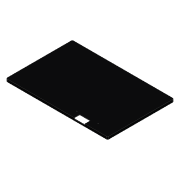
# Autodesk Inventor part: printer floor plate
Saved by Autodesk Inventor 2015 (Build 190159000, 159)
## iProperties
Created: 2018-06-07
Part Number: printer floor plate
Material: Generic
Document SubType Name: Modeling
Designer: Ghassan Yusuf
Density: 1 g/cm^3
Appearance: Default(1)
Author: Ghassan Yusuf
Autodesk Inventor part; units mm, degrees
ref_plane "YZ Plane" through (0, 0, 0) normal (1, 0, 0) x (0, 1, 0)
ref_plane "XZ Plane" through (0, 0, 0) normal (0, 1, 0) x (-1, 0, 0)
ref_plane "XY Plane" through (0, 0, 0) normal (0, 0, 1) x (1, 0, 0)
sketch "Sketch1" plane through (0, 0, 0) normal (0, 0, 1) x (1, 0, 0)
  line L0 (-236.677, 154.5) -> (236.677, 154.5)
  line L1 (236.677, 154.5) -> (236.677, -154.5)
  line L2 (236.677, -154.5) -> (-236.677, -154.5)
  line L3 (-236.677, -154.5) -> (-236.677, 154.5)
  point P0 (0, 0)
  point P1 (0, 154.5)
  point P2 (-236.677, 0)
  dimension "d0" = 473.354
  dimension "d1" = 309
  constraints: 8 end point, 2 midpoint, 2 parallel, 1 horizontal, 1 horizontal alignment, 1 perpendicular, 1 vertical alignment
  measures "d0" distance of L1.end L2.end
  measures "d1" distance of L0.end L1.end
extrude "Extrusion1" add sketch "Sketch1" along normal blind 2
sketch "Sketch2" plane through (0, 0, 2) normal (0, 0, 1) x (1, 0, 0)
  line L0 (-236.677, 154.5) -> (236.677, 154.5)
  line L1 (236.677, 154.5) -> (236.677, -154.5)
  line L2 (236.677, -154.5) -> (-236.677, -154.5)
  line L3 (-236.677, -154.5) -> (-236.677, 154.5)
  line L4 (-234.677, 152.5) -> (234.677, 152.5)
  line L5 (234.677, 152.5) -> (234.677, -152.5)
  line L6 (234.677, -152.5) -> (-234.677, -152.5)
  line L7 (-234.677, -152.5) -> (-234.677, 152.5)
  point P0 (0, 0)
  dimension "d4" = 2
  constraints: 16 end point, 4 parallel, 2 perpendicular, 1 horizontal, 3 other
  measures "d4" distance between parallel lines of L3 L7
extrude "Extrusion2" add sketch "Sketch2" along normal blind 10
fillet "Fillet1" radius 5 8 edges at (236.677, -154.5, 6) (234.677, -152.5, 7) (-236.677, -154.5, 6) (-234.677, -152.5, 7) (-234.677, 152.5, 7) (236.677, 154.5, 6) (234.677, 152.5, 7) (-236.677, 154.5, 6)
sketch "Sketch4" plane through (0, 0, 0) normal (0, 0, -1) x (-1, 0, 0)
  line L0 (-231.677, -154.5) -> (231.677, -154.5)
  line L1 (236.677, -149.5) -> (236.677, 149.5)
  line L2 (-80.477, 154.5) -> (-130.477, 154.5)
  line L3 (-130.477, 154.5) -> (-130.477, 128.5)
  line L4 (-130.477, 128.5) -> (-80.477, 128.5)
  line L5 (-80.477, 128.5) -> (-80.477, 154.5)
  line L6 (231.677, 154.5) -> (-231.677, 154.5) projected
  line L7 (-236.677, 149.5) -> (-236.677, -149.5) projected
  circle A0 centre (-60.807, 122.34) radius 1.5
  circle A1 centre (-160.677, 122.34) radius 1.5
  point P0 (0, 0)
  point P1 (0, 0)
  dimension "d24" = 50
  dimension "d25" = 106.2
  dimension "d26" = 3
  dimension "d27" = 3
  dimension "d28" = 32.16
  dimension "d29" = 99.87
  dimension "d30" = 76
  dimension "d33" = 26
  constraints: 12 end point, 2 centre point, 2 parallel, 1 collinear, 1 horizontal, 1 horizontal alignment, 1 perpendicular
  measures "d24" distance between parallel lines of L3 L5
  measures "d25" distance between parallel lines of L7 L3
  measures "d26" diameter of A0
  measures "d27" diameter of A1
  measures "d28" distance from line of A1.centre L6
  measures "d29" distance of A1.centre A0.centre
  measures "d30" distance from line of L7 A1.centre
  measures "d33" distance between parallel lines of L2 L4
extrude "Extrusion4" cut sketch "Sketch4" against normal blind 5
fillet "Fillet2" radius 3 4 edges at (80.477, 128.5, 1) (130.477, 128.5, 1) (130.477, 153.5, 5) (80.477, 153.5, 5)
body "Solid1"
